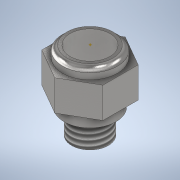
# Autodesk Inventor part: entrada_manguera_alicat_flujo
Saved by Autodesk Inventor 2022 (Build 260153000, 153)
## iProperties
Created: 2022-11-15
Part Number: entrada_manguera_alicat_flujo
Material: Generic
Document SubType Name: Modeling
Designer: ferna
Density: 1 g/cm^3
Appearance: Galvanized
Author: ferna
Autodesk Inventor part; units mm, degrees
ref_plane "YZ Plane" through (0, 0, 0) normal (1, 0, 0) x (0, 1, 0)
ref_plane "XZ Plane" through (0, 0, 0) normal (0, 1, 0) x (-1, 0, 0)
ref_plane "XY Plane" through (0, 0, 0) normal (0, 0, 1) x (1, 0, 0)
sketch "Sketch1" plane through (0, 0, 0) normal (0, 1, 0) x (-1, 0, 0)
  circle A0 centre (0, 0) radius 6
  circle A1 centre (0, 0) radius 4.5
  dimension "d2" = 12
  dimension "d3" = 9
  constraints: 2 centre point, 2 coincident
  measures "d2" diameter of A0
  measures "d3" diameter of A1
extrude "Extrusion1" add sketch "Sketch1" along normal blind 8
sketch "Sketch2" plane through (0, 8, 0) normal (0, 1, 0) x (1, 0, 0)
  circle A0 centre (0, 0) radius 8.5
  circle A1 centre (0, 0) radius 4.5 projected
  dimension "d6" = 17
  constraints: 1 centre point, 1 coincident
  measures "d6" diameter of A0
extrude "Extrusion2" add sketch "Sketch2" along normal blind 4
sketch "Sketch3" plane through (0, 12, 0) normal (0, 1, 0) x (1, 0, 0)
  line L0 (0, 0) -> (-10, 0)
  line L1 (-10, 5.7735) -> (0, 11.547)
  line L2 (0, 11.547) -> (10, 5.7735)
  line L3 (10, 5.7735) -> (10, -5.7735)
  line L4 (10, -5.7735) -> (0, -11.547)
  line L5 (0, -11.547) -> (-10, -5.7735)
  line L6 (-10, -5.7735) -> (-10, 5.7735)
  circle A0 centre (0, 0) radius 6 projected
  dimension "d9" = 10
  constraints: 14 end point, 1 coincident, 1 horizontal, 1 midpoint, 13 other
  measures "d9" distance of L0.start L0.end
extrude "Extrusion3" add sketch "Sketch3" along normal blind 10
sketch "Sketch4" plane through (0, 22, 0) normal (0, 1, 0) x (1, 0, 0)
  circle A0 centre (0, 0) radius 9
  circle A1 centre (0, 0) radius 6.5
  dimension "d12" = 18
  dimension "d13" = 13
  constraints: 2 centre point, 2 coincident
  measures "d12" diameter of A0
  measures "d13" diameter of A1
extrude "Extrusion4" add sketch "Sketch4" along normal blind 2
sketch "Sketch5" plane through (0, 24, 0) normal (0, 1, 0) x (1, 0, 0)
  circle A0 centre (0, 0) radius 6.5
  circle A1 centre (0, 0) radius 6.5 projected
  circle A2 centre (0, 0) radius 7.5
  dimension "d16" = 15
  constraints: 2 centre point, 2 coincident
  measures "d16" diameter of A2
extrude "Extrusion5" add sketch "Sketch5" along normal blind 1.5
fillet "Fillet1" radius 1.5 1 edges at (-7.5, 24, 0)
sketch "Sketch6" plane through (0, 25.5, 0) normal (0, 1, 0) x (1, 0, 0)
  circle A0 centre (0, 0) radius 7.5 projected
  circle A1 centre (0, 0) radius 6.5
  constraints: 1 centre point, 1 coincident
extrude "Extrusion6" cut sketch "Sketch6" against normal blind 13.5 contours A1
thread "Thread1" size "M12x1.75" class "6g" standard "ANSI Metric M Profile" full length
sketch "Sketch7" plane through (0, 25.5, 0) normal (0, 1, 0) x (1, 0, 0)
  circle A0 centre (0, 0) radius 6.5 projected
body "Solid1"
